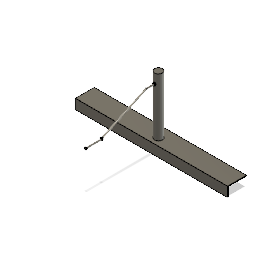
Coil winder v7 (Autodesk Fusion 360 archive; units mm, degrees)
design "base of coil winder"
Autodesk Fusion 360 part; units mm, degrees
sketch "Sketch1" plane through (0, 0, 0) normal (0, 1, 0) x (1, 0, 0)
  line L0 (-25, -15) -> (30, -15)
  line L1 (30, -15) -> (30, 95)
  line L2 (30, 95) -> (35, 95)
  line L3 (35, 95) -> (35, -20)
  line L4 (35, -20) -> (-25, -20)
  line L5 (-25, -20) -> (-25, -10)
  dimension "d1" = 55
  dimension "d2" = 110
  dimension "d3" = 10
  constraint horizontal L0
  constraint perpendicular L0 L1
  constraint perpendicular L1 L2
  constraint perpendicular L2 L3
  constraint perpendicular L1 L4
  measures "d1" distance of L0.start L0.end
  measures "d2" distance of L0.end L1.end
  measures "d3" distance of L4.end L5.end
extrude "Extrude1" add sketch "Sketch1" along normal blind 220 makes body 1
extrude "Extrude2" add 1 faces at (33.3333, 220, -20) along direction (0, 1, 0) blind 700 on bodies 1 bodies 1
move_body "Move1" bodies 1 to x (0, 1, 0) y (-1, 0, 0) z (0, 0, 1) at (-25, 25, 0)
sketch "Sketch2" plane through (0, 0, 0) normal (0, 1, 0) x (1, 0, 0)
  line L0 (-25, 25, 0) -> (-487.5, 25, 60)
  line L1 (-25, 95) -> (-945, 95)
  line L2 (-25, -20) -> (-945, -20)
  circle A0 through (-463.5, 25, 60) (-499.5, 45.7846, 60) (-499.5, 4.2154, 60)
  dimension "d10" = 48
extrude "Extrude3" add sketch "Sketch2" along normal blind 350 contours A0 in plane through (0, 60, 0) normal (0, 1, 0) bodies 1
sketch "Sketch3" plane through (0, 0, 0) normal (0, 1, 0) x (1, 0, 0)
  line L0 (92.1996, -50, 349.9015) -> (-832.8004, -50, 349.9015)
  circle A0 through (-475.9676, -58.3699, 349.2396) (-490.2452, -50.1268, 349.2396) (-490.2452, -66.6131, 349.2396)
  line L1 (-485.486, -58.3699, 349.2396) -> (-485.486, -330.2623, 222.4541)
  dimension "d14" = 300
pipe "Pipe1" add diameter 10 path "Sketch3" along L1 separate body makes body 2
mesh "Mesh1" [no effect]
sketch "Sketch4" plane through (0, 0, 0) normal (0, 1, 0) x (1, 0, 0)
  line L0 (-200, -75) -> (-190, -75)
  line L1 (-190, -75) -> (-186.9098, -65.4894)
  line L2 (-186.9098, -65.4894) -> (-195, -59.6116)
  line L3 (-195, -59.6116) -> (-203.0902, -65.4894)
  line L4 (-203.0902, -65.4894) -> (-200, -75)
  line L5 (-200, -75) -> (-199.9999, -75) construction
  point P0 (-195, -68.1181)
  dimension "d19" = 10
  dimension "d20" = 0
  constraint horizontal L5
  measures "d19" distance of L0.start L0.end
  measures "d20" angle of L0 L5
extrude "Extrude4" add sketch "Sketch4" along normal blind 5 separate body makes body 3
move_body "Move2" bodies 3 to x (1, 0, 0) y (0, 0, 1) z (0, -1, 0) at (-291.1877, 422.9533, -1.8062)
copy_body "CopyPasteBodies1" bodies 3 makes body 4
move_body "Move3" bodies 4 to x (1, 0, 0) y (0, 1, 0) z (0, 0, 1) at (0, 0, 4.8907)
sketch "Sketch5" plane through (0, 0, 0) normal (1, 0, 0) x (0, 0, -1)
  line L0 (-55.679, 354.3286, -485.449) -> (-10.679, 354.3286, -485.449)
pipe "Pipe2" add diameter 10 path "Sketch5" along L0 separate body makes body 5
move_body "Move4" bodies 5 to x (1, 0, 0) y (0, 1, 0) z (0, 0, 1) at (0, 0, -5)
move_body "Move5" bodies 2 to x (1, 0, 0) y (0, 1, 0) z (0, 0, 1) at (-0.2894, 5.0937, -8.6585)
move_body "Move6" bodies 2 to x (1, 0, 0) y (0, 1, 0) z (0, 0, 1) at (-0.7074, 0.2254, -1.1268)
copy_body "CopyPasteBodies2" bodies 3 makes body 6
move_body "Move7" bodies 6 to x (1, 0, 0) y (0, 0.906308, 0.422618) z (0, -0.422618, 0.906308) at (0, -94.1764, 170.2547)
copy_body "CopyPasteBodies3" bodies 6 makes body 7
move_body "Move8" bodies 7 to x (1, 0, 0) y (0, 0.965926, -0.258819) z (0, 0.258819, 0.965926) at (0, -74.2108, 67.6515)
sketch "Sketch6" plane through (0, 0, 0) normal (1, 0, 0) x (0, 0, -1)
  line L0 (-325, 225) -> (-425, 225)
  dimension "d27" = 100
  constraint horizontal L0
  measures "d27" distance of L0.start L0.end
pipe "Pipe3" add diameter 10 path "Sketch6" along L0 separate body makes body 8
move_face "MoveFace1" to x (1, 0, 0) y (0, 1, 0) z (0, 0, 1) at (0, 0, 5) 1 faces at (-4.6985, 223.2899, 358.3333) on bodies 8
move_face "MoveFace2" to x (1, 0, 0) y (0, 1, 0) z (0, 0, 1) at (-485.7512, 0, 46.2713) 1 faces at (-4.6985, 223.2899, 358.3333) on bodies 8
move_body "Move9" bodies 8 to x (1, 0, 0) y (0, 1, 0) z (0, 0, 1) at (0, 0, -10)
copy_body "CopyPasteBodies4" bodies 3 makes body 9
move_body "Move10" bodies 9 to x (1, 0, 0) y (0, 1, 0) z (0, 0, 1) at (-10.3716, -134.6755, 414.1823)
move_body "Move11" bodies 9 to x (1, 0, 0) y (0, 1, 0) z (0, 0, 1) at (9.9809, 4.2002, 0.2193)
